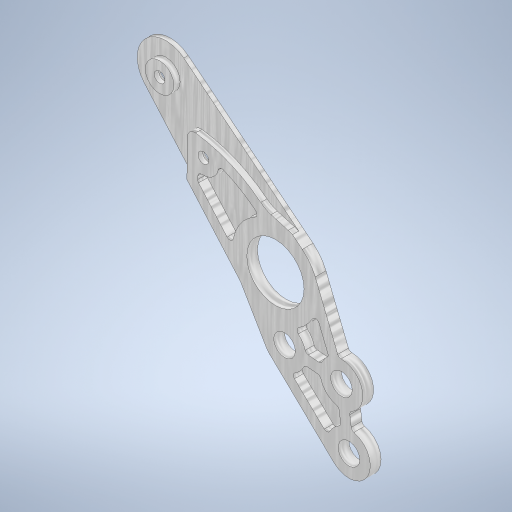
# Autodesk Inventor part: アーム 中間節(ミラー)
Saved by Autodesk Inventor 2023 (Build 270158000, 158)
## iProperties
Created: 2020-05-13
Part Number: アーム 中間節(ミラー)
Material: アルミニウム 7075
Document SubType Name: Modeling
Designer: mozar
Density: 2.81 g/cm^3
Appearance: サテン - ブラシ仕上げ 重厚
Author: mozar
Autodesk Inventor part; units mm, degrees
ref_plane "YZ Plane" through (0, 0, 0) normal (1, 0, 0) x (0, 1, 0)
ref_plane "XZ Plane" through (0, 0, 0) normal (0, 1, 0) x (-1, 0, 0)
ref_plane "XY Plane" through (0, 0, 0) normal (0, 0, 1) x (1, 0, 0)
sketch "スケッチ1" plane through (0, 0, 0) normal (0, 0, 1) x (1, 0, 0)
  circle A0 centre (89.1334, 60.2981) radius 8.025
  arc A1 (110.4927, 37.2495) -> (107.5312, 48.5254) centre (107.6371, 42.5263) ccw
  arc A2 (106.5859, 49.1517) -> (107.5312, 48.5254) centre (107.5135, 49.5253) ccw
  line L0 (106.5859, 49.1517) -> (100.2878, 64.7903)
  arc A3 (100.2878, 64.7903) -> (96.6592, 69.6769) centre (89.1334, 60.2981) ccw
  line L1 (96.6592, 69.6769) -> (61.7006, 97.7286)
  arc A4 (61.7006, 97.7286) -> (50.6268, 86.1987) centre (56.6782, 91.4695) ccw
  line L2 (50.6268, 86.1987) -> (79.2604, 53.3248)
  arc A5 (79.3697, 53.1725) -> (79.2604, 53.3248) centre (78.5063, 52.668) ccw
  line L3 (79.3697, 53.1725) -> (86.5144, 40.9457)
  arc A6 (86.5144, 40.9457) -> (87.5386, 39.6454) centre (91.6947, 43.9728) ccw
  line L4 (87.5386, 39.6454) -> (105.5692, 22.328)
  arc A7 (105.5692, 22.328) -> (111.1188, 32.4913) centre (109.7254, 26.6553) ccw
  arc A8 (110.3596, 33.3335) -> (111.1188, 32.4913) centre (111.3511, 33.464) ccw
  line L5 (110.3596, 33.3335) -> (109.9772, 36.2396)
  arc A9 (110.4927, 37.2495) -> (109.9772, 36.2396) centre (110.9687, 36.37) ccw
  circle A10 centre (68.955, 78.0364) radius 1.25
  circle A11 centre (109.7254, 26.6553) radius 3.025
  circle A12 centre (107.6371, 42.5263) radius 3.025
  circle A13 centre (91.6947, 43.9728) radius 3.025
  circle A14 centre (56.6782, 91.4695) radius 1.25
  arc A15 (83.1457, 72.8964) -> (83.5589, 72.581) centre (90.3437, 81.8972) ccw
  arc A16 (83.1457, 72.8964) -> (74.4673, 77.9243) centre (62.1124, 46.5952) ccw
  arc A17 (74.4673, 77.9243) -> (73.1203, 77.1926) centre (74.1004, 76.994) ccw
  arc A18 (68.4822, 73.8128) -> (73.1203, 77.1926) centre (68.955, 78.0364) ccw
  arc A19 (68.4822, 73.8128) -> (67.371, 72.8351) centre (68.3709, 72.819) ccw
  line L6 (67.371, 72.8351) -> (67.3568, 71.9495)
  arc A20 (67.3568, 71.9495) -> (67.6026, 71.2766) centre (68.3567, 71.9334) ccw
  line L7 (67.6026, 71.2766) -> (75.5898, 62.1066)
  arc A21 (75.5898, 62.1066) -> (77.3258, 62.5741) centre (76.3438, 62.7634) ccw
  arc A22 (83.4434, 70.8917) -> (77.3258, 62.5741) centre (89.1334, 60.2981) ccw
  arc A23 (83.4434, 70.8917) -> (83.5589, 72.581) centre (82.9702, 71.7727) ccw
  arc A24 (97.4697, 45.6005) -> (95.5411, 48.5777) centre (91.6947, 43.9728) ccw
  arc A25 (97.4697, 45.6005) -> (98.3419, 44.8759) centre (98.4322, 45.8718) ccw
  line L8 (98.3419, 44.8759) -> (101.261, 44.611)
  arc A26 (101.261, 44.611) -> (102.2493, 45.1668) centre (101.3514, 45.6069) ccw
  arc A27 (103.6511, 47.011) -> (102.2493, 45.1668) centre (107.6371, 42.5263) ccw
  arc A28 (103.6511, 47.011) -> (103.9749, 47.6045) centre (102.9868, 47.7585) ccw
  line L9 (103.9749, 47.6045) -> (101.3375, 54.1532)
  arc A29 (101.3375, 54.1532) -> (99.5442, 54.2801) centre (100.4099, 53.7796) ccw
  arc A30 (95.641, 50.1861) -> (99.5442, 54.2801) centre (89.1334, 60.2981) ccw
  arc A31 (95.641, 50.1861) -> (95.5411, 48.5777) centre (96.1822, 49.3452) ccw
  circle A32 centre (89.1334, 60.2981) radius 8.025
  arc A33 (110.4927, 37.2495) -> (107.5312, 48.5254) centre (107.6371, 42.5263) ccw
  arc A34 (110.4927, 37.2495) -> (109.9772, 36.2396) centre (110.9687, 36.37) ccw
  line L10 (109.9772, 36.2396) -> (110.3596, 33.3335)
  arc A35 (110.3596, 33.3335) -> (111.1188, 32.4913) centre (111.3511, 33.464) ccw
  arc A36 (105.5692, 22.328) -> (111.1188, 32.4913) centre (109.7254, 26.6553) ccw
  line L11 (105.5692, 22.328) -> (87.5386, 39.6454)
  arc A37 (86.5144, 40.9457) -> (87.5386, 39.6454) centre (91.6947, 43.9728) ccw
  line L12 (86.5144, 40.9457) -> (79.3697, 53.1725)
  arc A38 (79.3697, 53.1725) -> (79.2604, 53.3248) centre (78.5063, 52.668) ccw
  line L13 (79.2604, 53.3248) -> (64.3325, 70.4633)
  line L14 (64.3325, 70.4633) -> (64.5025, 81.0256)
  arc A39 (66.7554, 82.9773) -> (64.5025, 81.0256) centre (66.5022, 80.9934) ccw
  arc A40 (85.0194, 75.2394) -> (66.7554, 82.9773) centre (62.1124, 46.5952) ccw
  arc A41 (85.0194, 75.2394) -> (87.9169, 73.7249) centre (90.3437, 81.8972) ccw
  line L15 (87.9169, 73.7249) -> (92.6989, 72.3049)
  arc A42 (93.9266, 71.8696) -> (92.6989, 72.3049) centre (89.1334, 60.2981) ccw
  line L16 (93.9266, 71.8696) -> (96.6592, 69.6769)
  arc A43 (100.2878, 64.7903) -> (96.6592, 69.6769) centre (89.1334, 60.2981) ccw
  line L17 (100.2878, 64.7903) -> (106.5859, 49.1517)
  arc A44 (106.5859, 49.1517) -> (107.5312, 48.5254) centre (107.5135, 49.5253) ccw
  line L18 (107.3853, 32.9421) -> (107.0029, 35.8482)
  arc A45 (107.0029, 35.8482) -> (106.2437, 36.6904) centre (106.0114, 35.7177) ccw
  arc A46 (101.8621, 40.8987) -> (106.2437, 36.6904) centre (107.6371, 42.5263) ccw
  arc A47 (101.8621, 40.8987) -> (100.9899, 41.6233) centre (100.8996, 40.6274) ccw
  line L19 (100.9899, 41.6233) -> (98.0708, 41.8881)
  arc A48 (98.0708, 41.8881) -> (97.0825, 41.3323) centre (97.9804, 40.8922) ccw
  arc A49 (94.6542, 38.7535) -> (97.0825, 41.3323) centre (91.6947, 43.9728) ccw
  arc A50 (94.6542, 38.7535) -> (94.4548, 37.1624) centre (95.1475, 37.8836) ccw
  line L20 (94.4548, 37.1624) -> (102.8092, 29.1384)
  arc A51 (102.8092, 29.1384) -> (104.391, 29.4019) centre (103.5019, 29.8597) ccw
  arc A52 (106.8698, 31.9322) -> (104.391, 29.4019) centre (109.7254, 26.6553) ccw
  arc A53 (106.8698, 31.9322) -> (107.3853, 32.9421) centre (106.3938, 32.8117) ccw
  circle A54 centre (107.6371, 42.5263) radius 3.025
  circle A55 centre (68.955, 78.0364) radius 1.25
  circle A56 centre (91.6947, 43.9728) radius 3.025
  circle A57 centre (109.7254, 26.6553) radius 3.025
  line L21 (61.7006, 97.7286) -> (93.9266, 71.8696)
  arc A58 (93.9266, 71.8696) -> (92.6989, 72.3049) centre (89.1334, 60.2981) ccw
  line L22 (87.9169, 73.7249) -> (92.6989, 72.3049)
  arc A59 (85.0194, 75.2394) -> (87.9169, 73.7249) centre (90.3437, 81.8972) ccw
  arc A60 (85.0194, 75.2394) -> (66.7554, 82.9773) centre (62.1124, 46.5952) ccw
  arc A61 (66.7554, 82.9773) -> (64.5025, 81.0256) centre (66.5022, 80.9934) ccw
  line L23 (64.3325, 70.4633) -> (64.5025, 81.0256)
  line L24 (64.3325, 70.4633) -> (50.6268, 86.1987)
  arc A62 (61.7006, 97.7286) -> (50.6268, 86.1987) centre (56.6782, 91.4695) ccw
  circle A63 centre (56.6782, 91.4695) radius 4
  point P0 (0, 0)
  point P1 (0, 0)
  constraints: 104 point on circle, 64 centre point, 50 end point, 232 other
extrude "押し出し1" add sketch "スケッチ1" against normal blind 3 contours A9 L5 A8 A7 L4 A6 L3 A5 L2 L14 A39 A40 A41 L15 A42 L1 A3 L0 A2 A1 | A42 L15 A41 A40 A39 L14 L2 A4 L1 | A15 A23 A22 A21 L7 A20 L6 A19 A18 A17 A16 | A24 A31 A30 A29 L9 A28 A27 A26 L8 A25 | A53 A52 A51 L20 A50 A49 A48 L19 A47 A46 A45 L18 | A63
extrude "押し出し2" cut sketch "スケッチ1" against normal blind 2 contours A42 L15 A41 A40 A39 L14 L2 A4 L1
extrude "押し出し3" cut sketch "スケッチ1" against normal blind 2.5 contours A15 A23 A22 A21 L7 A20 L6 A19 A18 A17 A16 | A24 A31 A30 A29 L9 A28 A27 A26 L8 A25 | A53 A52 A51 L20 A50 A49 A48 L19 A47 A46 A45 L18
hole "穴1" at (68.955, 78.0364, 0) at (56.6782, 91.4695, 0) direction (0, 0, -1) diameter 3 depth 12 tip angle 118
sketch "スケッチ2" plane through (0, 0, -2) normal (0, 0, 1) x (1, 0, 0)
  circle A0 centre (68.955, 78.0364) radius 1.5 projected
  circle A1 centre (56.6782, 91.4695) radius 1.5 projected
  arc A2 (94.6542, 38.7535) -> (94.4548, 37.1624) centre (95.1475, 37.8836) ccw projected
  line L0 (94.4548, 37.1624) -> (102.8092, 29.1384) projected
  arc A3 (102.8092, 29.1384) -> (104.391, 29.4019) centre (103.5019, 29.8597) ccw projected
  arc A4 (106.8698, 31.9322) -> (104.391, 29.4019) centre (109.7254, 26.6553) ccw projected
  arc A5 (106.8698, 31.9322) -> (107.3853, 32.9421) centre (106.3938, 32.8117) ccw projected
  line L1 (107.3853, 32.9421) -> (107.0029, 35.8482) projected
  arc A6 (107.0029, 35.8482) -> (106.2437, 36.6904) centre (106.0114, 35.7177) ccw projected
  arc A7 (101.8621, 40.8987) -> (106.2437, 36.6904) centre (107.6371, 42.5263) ccw projected
  arc A8 (101.8621, 40.8987) -> (100.9899, 41.6233) centre (100.8996, 40.6274) ccw projected
  line L2 (100.9899, 41.6233) -> (98.0708, 41.8881) projected
  arc A9 (98.0708, 41.8881) -> (97.0825, 41.3323) centre (97.9804, 40.8922) ccw projected
  arc A10 (94.6542, 38.7535) -> (97.0825, 41.3323) centre (91.6947, 43.9728) ccw projected
  arc A11 (95.641, 50.1861) -> (95.5411, 48.5777) centre (96.1822, 49.3452) ccw projected
  arc A12 (97.4697, 45.6005) -> (95.5411, 48.5777) centre (91.6947, 43.9728) ccw projected
  arc A13 (97.4697, 45.6005) -> (98.3419, 44.8759) centre (98.4322, 45.8718) ccw projected
  line L3 (98.3419, 44.8759) -> (101.261, 44.611) projected
  arc A14 (101.261, 44.611) -> (102.2493, 45.1668) centre (101.3514, 45.6069) ccw projected
  arc A15 (103.6511, 47.011) -> (102.2493, 45.1668) centre (107.6371, 42.5263) ccw projected
  arc A16 (103.6511, 47.011) -> (103.9749, 47.6045) centre (102.9868, 47.7585) ccw projected
  line L4 (103.9749, 47.6045) -> (101.3375, 54.1532) projected
  arc A17 (101.3375, 54.1532) -> (99.5442, 54.2801) centre (100.4099, 53.7796) ccw projected
  arc A18 (95.641, 50.1861) -> (99.5442, 54.2801) centre (89.1334, 60.2981) ccw projected
  line L5 (67.371, 72.8351) -> (67.3568, 71.9495) projected
  arc A19 (67.3568, 71.9495) -> (67.6026, 71.2766) centre (68.3567, 71.9334) ccw projected
  line L6 (67.6026, 71.2766) -> (75.5898, 62.1066) projected
  arc A20 (75.5898, 62.1066) -> (77.3258, 62.5741) centre (76.3438, 62.7634) ccw projected
  arc A21 (83.4434, 70.8917) -> (77.3258, 62.5741) centre (89.1334, 60.2981) ccw projected
  arc A22 (83.4434, 70.8917) -> (83.5589, 72.581) centre (82.9702, 71.7727) ccw projected
  arc A23 (83.1457, 72.8964) -> (83.5589, 72.581) centre (90.3437, 81.8972) ccw projected
  arc A24 (83.1457, 72.8964) -> (74.4673, 77.9243) centre (62.1124, 46.5952) ccw projected
  arc A25 (74.4673, 77.9243) -> (73.1203, 77.1926) centre (74.1004, 76.994) ccw projected
  arc A26 (68.4822, 73.8128) -> (73.1203, 77.1926) centre (68.955, 78.0364) ccw projected
  arc A27 (68.4822, 73.8128) -> (67.371, 72.8351) centre (68.3709, 72.819) ccw projected
  circle A28 centre (56.6782, 91.4695) radius 4 projected
  line L7 (64.3325, 70.4633) -> (64.5025, 81.0256) projected
  arc A29 (66.7554, 82.9773) -> (64.5025, 81.0256) centre (66.5022, 80.9934) ccw projected
  arc A30 (85.0194, 75.2394) -> (66.7554, 82.9773) centre (62.1124, 46.5952) ccw projected
  arc A31 (85.0194, 75.2394) -> (87.9169, 73.7249) centre (90.3437, 81.8972) ccw projected
  line L8 (87.9169, 73.7249) -> (92.6989, 72.3049) projected
  arc A32 (93.9266, 71.8696) -> (92.6989, 72.3049) centre (89.1334, 60.2981) ccw projected
  line L9 (61.7006, 97.7286) -> (93.9266, 71.8696) projected
  arc A33 (61.7006, 97.7286) -> (50.6268, 86.1987) centre (56.6782, 91.4695) ccw projected
  line L10 (64.3325, 70.4633) -> (50.6268, 86.1987) projected
  line L11 (79.2604, 53.3248) -> (64.3325, 70.4633) projected
  arc A34 (79.3697, 53.1725) -> (79.2604, 53.3248) centre (78.5063, 52.668) ccw projected
  line L12 (86.5144, 40.9457) -> (79.3697, 53.1725) projected
  arc A35 (86.5144, 40.9457) -> (87.5386, 39.6454) centre (91.6947, 43.9728) ccw projected
  line L13 (105.5692, 22.328) -> (87.5386, 39.6454) projected
  arc A36 (105.5692, 22.328) -> (111.1188, 32.4913) centre (109.7254, 26.6553) ccw projected
  arc A37 (110.3596, 33.3335) -> (111.1188, 32.4913) centre (111.3511, 33.464) ccw projected
  line L14 (109.9772, 36.2396) -> (110.3596, 33.3335) projected
  arc A38 (110.4927, 37.2495) -> (109.9772, 36.2396) centre (110.9687, 36.37) ccw projected
  arc A39 (110.4927, 37.2495) -> (107.5312, 48.5254) centre (107.6371, 42.5263) ccw projected
  arc A40 (106.5859, 49.1517) -> (107.5312, 48.5254) centre (107.5135, 49.5253) ccw projected
  line L15 (100.2878, 64.7903) -> (106.5859, 49.1517) projected
  arc A41 (100.2878, 64.7903) -> (96.6592, 69.6769) centre (89.1334, 60.2981) ccw projected
  line L16 (93.9266, 71.8696) -> (96.6592, 69.6769) projected
  circle A42 centre (89.1334, 60.2981) radius 8.025 projected
  circle A43 centre (109.7254, 26.6553) radius 3.025 projected
  circle A44 centre (107.6371, 42.5263) radius 3.025 projected
  circle A45 centre (91.6947, 43.9728) radius 3.025 projected
  point P0 (0, 0)
extrude "押し出し4" add sketch "スケッチ2" along normal blind 0.25 contours L10 A33 L9 A32 L8 A31 A30 A29 L7
chamfer "面取り1" distance 1.75 angle 45 2 edges at (68.955, 79.5364, -3) (56.6782, 92.9695, -3)
